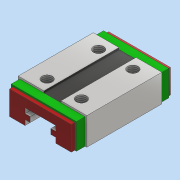
# Autodesk Inventor part: Wózel MGN9C
Saved by Autodesk Inventor 2018 (Build 220112000, 112)
## iProperties
Created: 2019-01-23
Part Number: Wózel MGN9C
Material: Ogólny
Document SubType Name: Modeling
Designer: Dawid
Density: 1 g/cm^3
Appearance: Aluminium — ciemne
Author: Dawid
Autodesk Inventor part; units mm, degrees
ref_plane "YZ Plane" through (0, 0, 0) normal (1, 0, 0) x (0, 1, 0)
ref_plane "XZ Plane" through (0, 0, 0) normal (0, 1, 0) x (-1, 0, 0)
ref_plane "XY Plane" through (0, 0, 0) normal (0, 0, 1) x (1, 0, 0)
sketch "Szkic1" plane through (0, 0, 0) normal (0, 0, 1) x (1, 0, 0)
  line L0 (0, 0) -> (10, 0)
  line L1 (10, 0) -> (10, 28.9)
  line L2 (10, 28.9) -> (-10, 28.9)
  line L3 (-10, 28.9) -> (-10, 0)
  line L4 (-10, 0) -> (10, 0)
  dimension "d1" = 28.9
  dimension "d2" = 20
  constraints: 10 end point, 4 perpendicular, 1 horizontal, 1 point on line
  measures "d1" distance of L0.end L1.end
  measures "d2" distance of L1.end L2.end
extrude "Wyciągnięcie proste1" add sketch "Szkic1" along normal blind 8
sketch "Szkic2" plane through (-10, 0, 0) normal (0, -1, 0) x (1, 0, 0)
  line L0 (0, 0) -> (20, 0)
  line L1 (20, 0) -> (20, 8)
  line L2 (0, 8) -> (20, 8)
  line L3 (0, 0) -> (0, 8)
  line L4 (14.5, 4.5) -> (5.5, 4.5)
  line L5 (14.5, 4.5) -> (14.5, 3)
  line L6 (14.5, 3) -> (13, 3)
  line L7 (13, 3) -> (13, 1.5)
  line L8 (13, 1.5) -> (14.5, 1.5)
  line L9 (5.5, 4.5) -> (5.5, 3)
  line L10 (5.5, 3) -> (7, 3)
  line L11 (7, 3) -> (7, 1.5)
  line L12 (7, 1.5) -> (5.5, 1.5)
  line L13 (5.5, 4.5) -> (5.5, 3)
  line L14 (5.5, 1.5) -> (5.5, 0)
  line L15 (14.5, 0) -> (14.5, 1.5)
  line L16 (14.5, 3) -> (14.5, 4.5)
  constraints: 34 end point, 2 point on line
extrude "Wyciągnięcie proste2" cut sketch "Szkic2" against normal up to next contours L14 L12 L11 L10 L9 L4 L5 L6 L7 L8 L15 L0
sketch "Szkic3" plane through (0, 0, 8) normal (0, 0, 1) x (1, 0, 0)
  line L0 (10, 0) -> (10, 28.9)
  line L1 (10, 28.9) -> (-10, 28.9)
  line L2 (-10, 28.9) -> (-10, 0)
  line L3 (-10, 0) -> (10, 0)
  line L4 (10, 28.9) -> (-10, 0)
  line L5 (10, 28.9) -> (-10, 28.9)
  line L6 (10, 0) -> (-10, 28.9)
  line L7 (-10, 28.9) -> (0, 14.45)
  line L8 (0, 14.45) -> (0, 6.95)
  line L9 (0, 6.95) -> (5, 6.95)
  line L10 (5, 6.95) -> (5, 21.95)
  line L11 (3, 0) -> (3, 28.9)
  line L12 (5, 21.95) -> (-5, 21.95)
  line L13 (-5, 21.95) -> (-5, 6.95)
  line L14 (-5, 6.95) -> (0, 6.95)
  line L15 (-3, 0) -> (-3, 28.9)
  circle A0 centre (5, 21.95) radius 1.5
  circle A1 centre (5, 6.95) radius 1.5
  circle A2 centre (-5, 21.95) radius 1.5
  circle A3 centre (-5, 6.95) radius 1.5
  point P0 (0, 0)
  dimension "d23" = 10
  dimension "d24" = 15
  dimension "d25" = 3
  dimension "d26" = 3
  dimension "d27" = 3
  dimension "d28" = 3
  constraints: 32 end point, 4 centre point, 4 coincident, 1 midpoint, 1 point on line
  measures "d23" distance between parallel lines of L13 L10
  measures "d24" distance of L9.end L10.end
  measures "d25" diameter of A0
  measures "d26" diameter of A1
  measures "d27" diameter of A2
  measures "d28" diameter of A3
extrude "Wyciągnięcie proste3" cut sketch "Szkic3" against normal blind 3 contours A1 L9 L10 L6 | L6 L10 A1 | A0 L10 L4 | L4 L10 L12 A0 | L10 L9 A1 L6 | L6 A1 L10 | L10 A0 L4 | L4 A0 L12 L10 | A3 L13 L4 | L4 L13 L14 A3 | L14 L13 L4 A3 | A2 L12 L13 L6 | L6 L13 A2 | A2 L6 L13 L12 | L13 A3 L4 | L6 A2 L13
thread "Gwint1" size "M3x0.5" class "6H" standard "ANSI Metric M Profile" full length
thread "Gwint2" size "M3x0.5" class "6H" standard "ANSI Metric M Profile" full length
thread "Gwint3" size "M3x0.5" class "6H" standard "ANSI Metric M Profile" full length
thread "Gwint4" size "M3x0.5" class "6H" standard "ANSI Metric M Profile" full length
sketch "Szkic4" plane through (0, 0, 8) normal (0, 0, 1) x (1, 0, 0)
  circle A0 centre (-5, 6.95) radius 1.5
  circle A1 centre (5, 6.95) radius 1.5
  circle A2 centre (5, 21.95) radius 1.5
  circle A3 centre (-5, 21.95) radius 1.5
  line L0 (10, 28.9) -> (-10, 28.9)
  line L1 (-10, 0) -> (10, 0)
  line L2 (-10, 0) -> (-10, 1)
  line L3 (-10, 1) -> (10, 1)
  line L4 (-10, 28.9) -> (-10, 27.9)
  line L5 (-10, 27.9) -> (10, 27.9)
  line L6 (-10, 28.9) -> (-10, 27.9)
  line L7 (-10, 1) -> (-10, 0)
  line L8 (10, 0) -> (10, 1)
  line L9 (10, 27.9) -> (10, 28.9)
  line L10 (10, 0) -> (10, 1)
  line L11 (10, 27.9) -> (10, 28.9)
  line L12 (-10, 28.9) -> (-10, 27.9)
  line L13 (-10, 1) -> (-10, 0)
  point P0 (0, 0)
  dimension "d39" = 1
  dimension "d40" = 1
  constraints: 28 end point, 7 centre point
  measures "d39" distance of L1.start L2.end
  measures "d40" distance of L0.end L4.end
extrude "Wyciągnięcie proste4" cut sketch "Szkic4" against normal blind 1 contours L9 L5 L4 L0 | L2 L3 L8 L1
sketch "Szkic5" plane through (10, 0, 0) normal (1, 0, 0) x (0, 0, -1)
  line L0 (-7, 1) -> (-7, 0) projected
  line L1 (0, 0) -> (-7, 0) projected
  line L2 (0, 0) -> (0, 28.9) projected
  line L3 (-7, 28.9) -> (-7, 27.9) projected
  line L4 (0, 28.9) -> (-7, 28.9) projected
  line L5 (-7, 1) -> (0, 1)
  line L6 (-7, 27.9) -> (0, 27.9)
  constraints: 4 end point, 2 point on line, 1 parallel, 1 perpendicular
extrude "Wyciągnięcie proste5" cut sketch "Szkic5" against normal blind 1
sketch "Szkic6" plane through (-10, 0, 0) normal (-1, 0, 0) x (0, 0, 1)
  line L0 (7, 27.9) -> (7, 28.9) projected
  line L1 (0, 28.9) -> (7, 28.9) projected
  line L2 (0, 28.9) -> (0, 0) projected
  line L3 (0, 0) -> (7, 0) projected
  line L4 (7, 0) -> (7, 1) projected
  line L5 (8, 27.9) -> (7, 27.9) projected
  line L6 (7, 27.9) -> (0, 27.9)
  line L7 (7, 1) -> (0, 1)
  constraints: 4 end point, 2 point on line, 1 parallel, 1 perpendicular
extrude "Wyciągnięcie proste6" cut sketch "Szkic6" against normal blind 1
sketch "Szkic7" plane through (0, 0, 8) normal (0, 0, 1) x (1, 0, 0)
  circle A0 centre (-5, 21.95) radius 1.5
  circle A1 centre (5, 21.95) radius 1.5
  circle A2 centre (5, 6.95) radius 1.5
  circle A3 centre (-5, 6.95) radius 1.5
  line L0 (-10, 1) -> (10, 1)
  line L1 (10, 27.9) -> (-10, 27.9)
  line L2 (10, 27.9) -> (10, 25.4)
  line L3 (10, 25.4) -> (-10, 25.4)
  line L4 (10, 1) -> (9, 1)
  line L5 (10, 1) -> (10, 3.5)
  line L6 (10, 3.5) -> (-10, 3.5)
  line L7 (10, 1) -> (10, 3.5)
  line L8 (10, 25.4) -> (10, 27.9)
  line L9 (10, 1) -> (10, 3.5)
  line L10 (10, 25.4) -> (10, 27.9)
  line L11 (-10, 27.9) -> (-10, 25.4)
  line L12 (-10, 3.5) -> (-10, 1)
  line L13 (-10, 27.9) -> (-10, 25.4)
  line L14 (-10, 3.5) -> (-10, 1)
  point P0 (0, 0)
  dimension "d47" = 2.5
  dimension "d48" = 2.5
  constraints: 30 end point, 7 centre point
  measures "d47" distance of L1.start L2.end
  measures "d48" distance of L0.end L5.end
extrude "Wyciągnięcie proste7" cut sketch "Szkic7" against normal blind 0.5 contours L12 L6 L5 L0 | L2 L3 L11 L1
sketch "Szkic8" plane through (-10, 1, 0) normal (-1, 0, 0) x (0, 0, 1)
  line L0 (7.5, 24.4) -> (7.5, 26.9) projected
  line L1 (7.5, 26.9) -> (0, 26.9) projected
  line L2 (7.5, 0) -> (7.5, 2.5) projected
  line L3 (0, 0) -> (7.5, 0) projected
  line L4 (0, 26.9) -> (0, 0) projected
  line L5 (7.5, 24.4) -> (0, 24.4)
  line L6 (7.5, 2.5) -> (7.5, 0) projected
  line L7 (7.5, 2.5) -> (0, 2.5)
  point P0 (0, -1)
  constraints: 4 end point, 2 perpendicular, 2 point on line
extrude "Wyciągnięcie proste8" cut sketch "Szkic8" against normal blind 0.5
sketch "Szkic9" plane through (10, 1, 0) normal (1, 0, 0) x (0, 0, -1)
  line L0 (-7.5, 2.5) -> (-7.5, 0) projected
  line L1 (-7.5, 0) -> (0, 0) projected
  line L2 (-7.5, 26.9) -> (-7.5, 24.4) projected
  line L3 (0, 26.9) -> (-7.5, 26.9) projected
  line L4 (0, 0) -> (0, 26.9) projected
  line L5 (0, 2.5) -> (-8, 2.5) projected
  line L6 (-7.5, 2.5) -> (0, 2.5)
  line L7 (-8, 24.4) -> (0, 24.4) projected
  line L8 (-7.5, 24.4) -> (0, 24.4)
  point P0 (0, -1)
  constraints: 4 end point, 1 collinear, 1 horizontal
extrude "Wyciągnięcie proste9" cut sketch "Szkic9" against normal blind 0.5
sketch "Szkic10" plane through (0, 0, 8) normal (0, 0, 1) x (1, 0, 0)
  line L0 (-10, 3.5) -> (10, 3.5) projected
  line L1 (10, 3.5) -> (10, 25.4) projected
  line L2 (10, 25.4) -> (-10, 25.4) projected
  line L3 (-10, 25.4) -> (-10, 3.5) projected
  circle A0 centre (-5, 21.95) radius 1.5 projected
  circle A1 centre (5, 21.95) radius 1.5 projected
  circle A2 centre (5, 6.95) radius 1.5 projected
  circle A3 centre (-5, 6.95) radius 1.5 projected
  line L4 (0, 3.5) -> (-2.5, 3.5)
  line L5 (-9.5, 3.5) -> (9.5, 3.5) projected
  line L6 (-2.5, 3.5) -> (-2.5, 25.4)
  line L7 (10, 25.4) -> (-10, 25.4) projected
  line L8 (-2.5, 25.4) -> (2.5, 25.4)
  line L9 (2.5, 25.4) -> (2.5, 3.5)
  line L10 (0, 3.5) -> (2.5, 3.5)
  point P0 (0, 0)
  dimension "d55" = 2.5
  dimension "d56" = 5
  constraints: 10 end point, 4 point on line, 2 perpendicular, 1 collinear, 1 midpoint
  measures "d55" distance of L4.start L4.end
  measures "d56" distance of L6.end L8.end
extrude "Wyciągnięcie proste10" cut sketch "Szkic10" against normal blind 0.6 contours L6 L2 L9 L0
